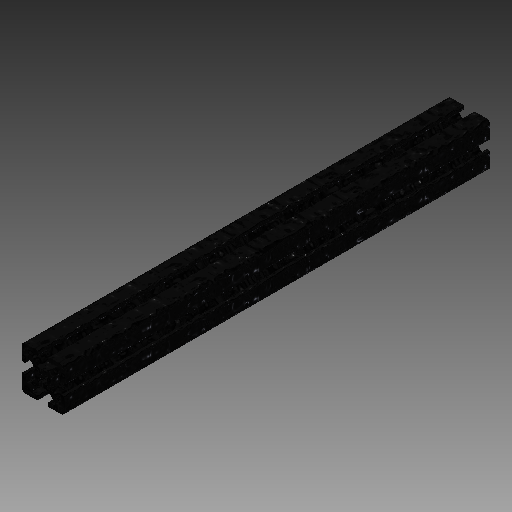
# Autodesk Inventor part: 1515-S
Saved by Autodesk Inventor 2019 (Build 230136000, 136)
## iProperties
Company: 80/20 Inc.
Created: 2013-09-06
Part Number: 1515-S
Material: Aluminum
Document SubType Name: Modeling
Density: 2.7 g/cm^3
Catalog Web Link: 8020.net
Vendor: 80/20 Inc.
Engineer: Ross Bowman
Appearance: Black
Author: Ross Bowman
Keywords: T-Slot, Extrusion, 80/20, 8020, Quick Frame, HT
Autodesk Inventor part; units mm, degrees
ref_plane "YZ Plane" through (0, 0, 0) normal (1, 0, 0) x (0, 1, 0)
ref_plane "XZ Plane" through (0, 0, 0) normal (0, 1, 0) x (-1, 0, 0)
ref_plane "Work Plane1" through (-293.8098, -15.875, -838.2) normal (0, 0, 1) x (1, 0, 0)
sketch "Sketch1" plane through (0, 0, 0) normal (0, 0, 1) x (1, 0, 0)
  arc A0 (4.2456, 2.6398) -> (2.6398, 4.2456) centre (3.5351, 3.5351) ccw
  line L0 (2.9729, 1.3564) -> (4.2456, 2.6398)
  arc A1 (2.9729, -1.3564) -> (2.9729, 1.3564) centre (0, 0) ccw
  line L1 (4.3433, -2.7269) -> (2.9729, -1.3564)
  arc A2 (2.7269, -4.3433) -> (4.3433, -2.7269) centre (3.5351, -3.5351) ccw
  line L2 (1.3564, -2.9729) -> (2.7269, -4.3433)
  arc A3 (-1.3564, -2.9729) -> (1.3564, -2.9729) centre (0, 0) ccw
  line L3 (-2.7269, -4.3433) -> (-1.3564, -2.9729)
  arc A4 (-4.3433, -2.7269) -> (-2.7269, -4.3433) centre (-3.5351, -3.5351) ccw
  line L4 (-2.9729, -1.3564) -> (-4.3433, -2.7269)
  arc A5 (-2.9729, 1.3564) -> (-2.9729, -1.3564) centre (0, 0) ccw
  line L5 (-4.3433, 2.7269) -> (-2.9729, 1.3564)
  arc A6 (-2.7269, 4.3433) -> (-4.3433, 2.7269) centre (-3.5351, 3.5351) ccw
  line L6 (-1.3564, 2.9729) -> (-2.7269, 4.3433)
  arc A7 (1.3564, 2.9729) -> (-1.3564, 2.9729) centre (0, 0) ccw
  line L7 (2.6398, 4.2456) -> (1.3564, 2.9729)
  arc A8 (16.5608, -4.064) -> (14.986, -5.6388) centre (16.5608, -5.6388) ccw
  line L8 (14.986, -5.6388) -> (14.986, -9.398)
  arc A9 (14.097, -10.287) -> (14.986, -9.398) centre (14.097, -9.398) ccw
  line L9 (14.097, -10.287) -> (13.5289, -10.287)
  arc A10 (12.9003, -10.0266) -> (13.5289, -10.287) centre (13.5289, -9.398) ccw
  line L10 (12.9003, -10.0266) -> (8.2608, -5.3872)
  arc A11 (6.8697, -2.0285) -> (8.2608, -5.3872) centre (11.6195, -2.0285) ccw
  line L11 (6.8697, -2.0285) -> (6.8697, 2.0285)
  arc A12 (8.2608, 5.3872) -> (6.8697, 2.0285) centre (11.6195, 2.0285) ccw
  line L12 (8.2608, 5.3872) -> (12.9003, 10.0266)
  arc A13 (13.5289, 10.287) -> (12.9003, 10.0266) centre (13.5289, 9.398) ccw
  line L13 (13.5289, 10.287) -> (14.097, 10.287)
  arc A14 (14.986, 9.398) -> (14.097, 10.287) centre (14.097, 9.398) ccw
  line L14 (14.986, 9.398) -> (14.986, 5.6388)
  arc A15 (14.986, 5.6388) -> (16.5608, 4.064) centre (16.5608, 5.6388) ccw
  line L15 (16.5608, 4.064) -> (17.4752, 4.064)
  arc A16 (17.4752, 4.064) -> (19.05, 5.6388) centre (17.4752, 5.6388) ccw
  line L16 (19.05, 5.6388) -> (19.05, 15.875)
  arc A17 (19.05, 15.875) -> (15.875, 19.05) centre (15.875, 15.875) ccw
  line L17 (15.875, 19.05) -> (5.6388, 19.05)
  arc A18 (5.6388, 19.05) -> (4.064, 17.4752) centre (5.6388, 17.4752) ccw
  line L18 (4.064, 17.4752) -> (4.064, 16.5608)
  arc A19 (4.064, 16.5608) -> (5.6388, 14.986) centre (5.6388, 16.5608) ccw
  line L19 (5.6388, 14.986) -> (9.398, 14.986)
  arc A20 (10.287, 14.097) -> (9.398, 14.986) centre (9.398, 14.097) ccw
  line L20 (10.287, 14.097) -> (10.287, 13.5289)
  arc A21 (10.0266, 12.9003) -> (10.287, 13.5289) centre (9.398, 13.5289) ccw
  line L21 (10.0266, 12.9003) -> (5.3872, 8.2608)
  arc A22 (2.0285, 6.8697) -> (5.3872, 8.2608) centre (2.0285, 11.6195) ccw
  line L22 (2.0285, 6.8697) -> (-2.0285, 6.8697)
  arc A23 (-5.3872, 8.2608) -> (-2.0285, 6.8697) centre (-2.0285, 11.6195) ccw
  line L23 (-5.3872, 8.2608) -> (-10.0266, 12.9003)
  arc A24 (-10.287, 13.5289) -> (-10.0266, 12.9003) centre (-9.398, 13.5289) ccw
  line L24 (-10.287, 13.5289) -> (-10.287, 14.097)
  arc A25 (-9.398, 14.986) -> (-10.287, 14.097) centre (-9.398, 14.097) ccw
  line L25 (-9.398, 14.986) -> (-5.6388, 14.986)
  arc A26 (-5.6388, 14.986) -> (-4.064, 16.5608) centre (-5.6388, 16.5608) ccw
  line L26 (-4.064, 16.5608) -> (-4.064, 17.4752)
  arc A27 (-4.064, 17.4752) -> (-5.6388, 19.05) centre (-5.6388, 17.4752) ccw
  line L27 (-5.6388, 19.05) -> (-15.875, 19.05)
  arc A28 (-15.875, 19.05) -> (-19.05, 15.875) centre (-15.875, 15.875) ccw
  line L28 (-19.05, 15.875) -> (-19.05, 5.6388)
  arc A29 (-19.05, 5.6388) -> (-17.4752, 4.064) centre (-17.4752, 5.6388) ccw
  line L29 (-17.4752, 4.064) -> (-16.5608, 4.064)
  arc A30 (-16.5608, 4.064) -> (-14.986, 5.6388) centre (-16.5608, 5.6388) ccw
  line L30 (-14.986, 5.6388) -> (-14.986, 9.398)
  arc A31 (-14.097, 10.287) -> (-14.986, 9.398) centre (-14.097, 9.398) ccw
  line L31 (-14.097, 10.287) -> (-13.5289, 10.287)
  arc A32 (-12.9003, 10.0266) -> (-13.5289, 10.287) centre (-13.5289, 9.398) ccw
  line L32 (-12.9003, 10.0266) -> (-8.2608, 5.3872)
  arc A33 (-6.8697, 2.0285) -> (-8.2608, 5.3872) centre (-11.6195, 2.0285) ccw
  line L33 (-6.8697, 2.0285) -> (-6.8697, -2.0285)
  arc A34 (-8.2608, -5.3872) -> (-6.8697, -2.0285) centre (-11.6195, -2.0285) ccw
  line L34 (-8.2608, -5.3872) -> (-12.9003, -10.0266)
  arc A35 (-13.5289, -10.287) -> (-12.9003, -10.0266) centre (-13.5289, -9.398) ccw
  line L35 (-13.5289, -10.287) -> (-14.097, -10.287)
  arc A36 (-14.986, -9.398) -> (-14.097, -10.287) centre (-14.097, -9.398) ccw
  line L36 (-14.986, -9.398) -> (-14.986, -5.6388)
  arc A37 (-14.986, -5.6388) -> (-16.5608, -4.064) centre (-16.5608, -5.6388) ccw
  line L37 (-16.5608, -4.064) -> (-17.4752, -4.064)
  arc A38 (-17.4752, -4.064) -> (-19.05, -5.6388) centre (-17.4752, -5.6388) ccw
  line L38 (-19.05, -5.6388) -> (-19.05, -15.875)
  arc A39 (-19.05, -15.875) -> (-15.875, -19.05) centre (-15.875, -15.875) ccw
  line L39 (-15.875, -19.05) -> (-5.6388, -19.05)
  arc A40 (-5.6388, -19.05) -> (-4.064, -17.4752) centre (-5.6388, -17.4752) ccw
  line L40 (-4.064, -17.4752) -> (-4.064, -16.5608)
  arc A41 (-4.064, -16.5608) -> (-5.6388, -14.986) centre (-5.6388, -16.5608) ccw
  line L41 (-5.6388, -14.986) -> (-9.398, -14.986)
  arc A42 (-10.287, -14.097) -> (-9.398, -14.986) centre (-9.398, -14.097) ccw
  line L42 (-10.287, -14.097) -> (-10.287, -13.5289)
  arc A43 (-10.0266, -12.9003) -> (-10.287, -13.5289) centre (-9.398, -13.5289) ccw
  line L43 (-10.0266, -12.9003) -> (-5.3872, -8.2608)
  arc A44 (-2.0285, -6.8697) -> (-5.3872, -8.2608) centre (-2.0285, -11.6195) ccw
  line L44 (-2.0285, -6.8697) -> (2.0285, -6.8697)
  arc A45 (5.3872, -8.2608) -> (2.0285, -6.8697) centre (2.0285, -11.6195) ccw
  line L45 (5.3872, -8.2608) -> (10.0266, -12.9003)
  arc A46 (10.287, -13.5289) -> (10.0266, -12.9003) centre (9.398, -13.5289) ccw
  line L46 (10.287, -13.5289) -> (10.287, -14.097)
  arc A47 (9.398, -14.986) -> (10.287, -14.097) centre (9.398, -14.097) ccw
  line L47 (9.398, -14.986) -> (5.6388, -14.986)
  arc A48 (5.6388, -14.986) -> (4.064, -16.5608) centre (5.6388, -16.5608) ccw
  line L48 (4.064, -16.5608) -> (4.064, -17.4752)
  arc A49 (4.064, -17.4752) -> (5.6388, -19.05) centre (5.6388, -17.4752) ccw
  line L49 (5.6388, -19.05) -> (15.875, -19.05)
  arc A50 (15.875, -19.05) -> (19.05, -15.875) centre (15.875, -15.875) ccw
  line L50 (19.05, -15.875) -> (19.05, -5.6388)
  arc A51 (19.05, -5.6388) -> (17.4752, -4.064) centre (17.4752, -5.6388) ccw
  line L51 (17.4752, -4.064) -> (16.5608, -4.064)
  constraints: 104 end point, 104 point on circle, 52 centre point
extrude "Extrusion1" add sketch "Sketch1" against normal blind 374.65
body "Solid1"
